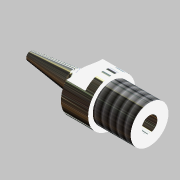
# Autodesk Inventor part: YTP-AP-E03-R1.0
Saved by Autodesk Inventor 2020.4 (Build 244396010, 396A)
## iProperties
Created: 2021-08-28
Part Number: YTP-AP-E03-R1.0
Material: Stahl
Document SubType Name: Modeling
Designer: Uwe Wieser
Mass: 0.0965333 g
Surface Area: 0.498236 cm^2
Volume: 0.0122972 cm^3
Density: 7.85 g/cm^3
Appearance: Chrom - poliert
Project: Airbrush
Description: HP-C Düse-0,3
Werkstoff: 1.4301
Author: Uwe Wieser
Autodesk Inventor part; units mm, degrees
sketch "Skizze1" plane through (0, 0, 0) normal (0, 0, 1) x (1, 0, 0)
  line L0 (-4.5575, 0) -> (5.2951, 0) projected
  line L1 (0, -0.25) -> (0, 1.5) projected
  line L2 (-3.15, 0) -> (-3.15, 0.225)
  line L3 (-3.15, 0.225) -> (-0.288, 0.583)
  line L4 (-3.15, 0.225) -> (-0.2657, 0.225) construction
  line L5 (-0.288, 0.583) -> (-0.288, 1.25)
  line L6 (-0.288, 1.25) -> (1.15, 1.25)
  line L7 (1.15, 1.25) -> (1.15, 1)
  line L8 (1.15, 1) -> (3.15, 1)
  line L9 (3.15, 1) -> (3.15, 0)
  arc A0 (3.8876, 1) -> (3.801, 0.95) centre (3.8876, 0.9) ccw
  arc A1 (3.2366, 0.95) -> (3.15, 1) centre (3.15, 0.9) ccw
  arc A2 (3.4322, 0.6112) -> (3.6054, 0.6112) centre (3.5188, 0.6612) ccw
  line L10 (3.4322, 0.6112) -> (3.2366, 0.95)
  line L11 (3.6054, 0.6112) -> (3.801, 0.95)
  line L12 (3.8876, 1) -> (3.15, 1)
  point P0 (0, 0)
  point P1 (3.1775, 0.57)
  dimension "d0" = 7.13
  dimension "d1" = 2
  dimension "d2" = 2.862
  dimension "d3" = 6.3
  dimension "d4" = 2
  dimension "d5" = 2.5
  dimension "d6" = 0.45
  dimension "d27" = 0.2
  dimension "d28" = 0.2
  dimension "d29" = 0.2
  dimension "d30" = 60
  constraints: 22 end point, 7 point on circle, 5 tangent, 4 perpendicular, 3 centre point, 3 point on line, 2 horizontal, 2 vertical, 1 equal length, 1 horizontal alignment, 1 symmetric about line
  measures "d0" angle of L4 L3
  measures "d1" distance of L7.end L8.end
  measures "d2" horizontal distance of L3.end L2.end
  measures "d3" distance of L2.start L9.end
  measures "d4" diameter of L8 L0
  measures "d5" diameter of L6 L0
  measures "d6" diameter of L2.end L0
  measures "d27" diameter of A0
  measures "d28" diameter of A1
  measures "d29" diameter of A2
  measures "d30" angle of L10 L11
revolve "Umdrehung1" add sketch "Skizze1" angle 360 about axis through (-10, 0, 0) along (1, 0, 0) contours L2 L3 L5 L6 L1 L0 | L1 L6 L7 L8 L9 L0
sketch "Skizze2" plane through (-0.288, 0, 0) normal (-1, 0, 0) x (0, 0, 1)
  circle A0 centre (0, 0) radius 0.583 projected
  circle A1 centre (0, 0) radius 1.25 projected
  circle A2 centre (0, 0) radius 1.25 projected
  line L0 (-0.8, -0.9605) -> (-0.8, 0.9605)
  line L1 (0, -1.75) -> (0, 1.75) projected
  line L2 (-1.75, 0) -> (1.75, 0) projected
  line L3 (0.8, -0.9605) -> (0.8, 0.9605)
  circle A3 centre (0, 0) radius 0.225 projected
  arc A4 (-0.8, 0.9605) -> (-0.8, -0.9605) centre (0, 0) ccw
  arc A5 (0.8, -0.9605) -> (0.8, 0.9605) centre (0, 0) ccw
  dimension "d10" = 1.6
  constraints: 4 end point, 4 point on circle, 2 centre point, 2 symmetric about line, 1 coincident, 1 parallel, 4 other
  measures "d10" distance of L3.end L0.end
extrude "Extrusion1" cut sketch "Skizze2" against normal blind 1 contours L3 A1 L2 | L2 A1 L3 | L2 A1 L0 | L0 A1 L2
fillet "Rundung1" radius 0.7 1 edges at (-0.288, -0.583, 0)
ref_plane "Arbeitsebene1" through (1.565, 0, 0) normal (1, 0, 0) x (0, 0, -1)
ref_plane "Arbeitsebene2" through (0, 0, 0) normal (0, 1, 0) x (-1, 0, 0)
sketch "Skizze4" plane through (0, 0, 0) normal (0, 1, 0) x (-1, 0, 0)
  line L0 (-3.15, 1) -> (-3.15, -1) projected
  line L1 (-3.15, 0.414) -> (3.15, 0.15)
  line L2 (3.15, 0.225) -> (3.15, -0.225) projected
  line L3 (4.41, 0) -> (-4.41, 0) projected
  line L4 (-3.15, 0.414) -> (-3.15, 0)
  line L5 (3.15, 0.15) -> (3.15, 0)
  point P0 (0, 0)
  dimension "d24" = 177.6
  dimension "d25" = 0.828
  constraints: 6 end point, 4 point on line, 2 midpoint
  measures "d24" angle of L3 L1
  measures "d25" diameter of L1.start L3
revolve "Umdrehung2" cut sketch "Skizze4" angle 360 about axis through (-10, 0, 0) along (1, 0, 0)
ref_plane "Arbeitsebene3" through (0, 0, 0) normal (0, 1, 0) x (-1, 0, 0)
ref_plane "Arbeitsebene4" through (1.15, 0, 0) normal (1, 0, 0) x (0, 1, 0)
sketch "Skizze7" plane through (1.15, 0, 0) normal (1, 0, 0) x (0, 1, 0)
  circle A0 centre (0, 0) radius 1
  circle A1 centre (0, 0) radius 0.3301
  dimension "d48" = 2
  constraints: 2 centre point, 2 coincident
  measures "d48" diameter of A0
extrude "Extrusion5" add sketch "Skizze7" along normal blind 0.45
ref_plane "Arbeitsebene5" through (0, 0, 0) normal (0, 0, 1) x (1, 0, 0)
sketch "Skizze8" plane through (0, 0, 0) normal (0, 0, 1) x (1, 0, 0)
  line L0 (-3.892, 0) -> (3.9838, 0)
  line L1 (-3.1473, 0.1581) -> (3.1494, 0.4137)
  line L2 (-3.1473, 0.1581) -> (-3.1473, 0)
  line L3 (3.1494, 0.4137) -> (3.1494, 0)
  line L4 (-3.1473, 0) -> (3.1494, 0)
  point P0 (0, 0)
  dimension "d56" = 0.3163
  dimension "d57" = 0.8275
  constraints: 10 end point, 2 perpendicular, 2 point on line, 1 collinear, 1 horizontal
  measures "d56" diameter of L1.start L0
  measures "d57" diameter of L1.end L0
revolve "Umdrehung3" cut sketch "Skizze8" angle 360 about axis through (-3.892, 0, 0) along (1, 0, 0)
thread "Gewinde2" size "M2x0.4" class "6g" standard "ISO Metric profile" length 10
